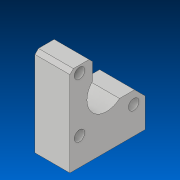
# Autodesk Inventor part: y-stepper-mount
Saved by Autodesk Inventor 2021 (Build 250183000, 183)
## iProperties
RuleStatus: InUse
Created: 2019-07-31
Part Number: y-stepper-mount
Material: Všeobecné
Document SubType Name: Modeling
Designer: Robert Turinský
Density: 1 g/cm^3
Appearance: Výchozí
Author: Robert Turinský
Autodesk Inventor part; units mm, degrees
ref_plane "XY Plane" through (0, 0, 0) normal (0, 0, 1) x (1, 0, 0)
sketch "Náčrt1" plane through (0, 0, 0) normal (0, 0, 1) x (1, 0, 0)
  line L0 (0, -49.6) -> (0, 14.1) projected
  line L1 (-71.6, 0) -> (163.6, 0) projected
  arc A0 (0.375, -4.0577) -> (-0.375, -4.0577) centre (0, 0) ccw
  arc A1 (120.375, -4.0577) -> (119.625, -4.0577) centre (120, 0) ccw
  line L2 (5, 5) -> (-5, 5)
  line L3 (-5, 5) -> (-8.1754, -0.5)
  line L4 (-8.1754, -0.5) -> (-35.5, -0.5)
  line L5 (-35.5, -0.5) -> (-38, -3)
  line L6 (-38, -3) -> (-38, -38)
  line L7 (-38, -38) -> (-35.5, -40.5)
  line L8 (-35.5, -40.5) -> (114, -40.5)
  line L9 (114, -40.5) -> (130, -24.5)
  line L10 (130, -24.5) -> (130, -3.6603)
  line L11 (130, -3.6603) -> (125, 5)
  line L12 (125, 5) -> (115, 5)
  line L13 (115, 5) -> (111.8246, -0.5)
  line L14 (111.8246, -0.5) -> (8.1754, -0.5)
  line L15 (8.1754, -0.5) -> (5, 5)
  circle A2 centre (87.45, -12.35) radius 2.65
  circle A3 centre (110.7, -35.6) radius 2.65
  circle A4 centre (-32.55, -12.35) radius 2.65
  circle A5 centre (-9.3, -35.6) radius 2.65
  line L16 (119.625, -4.0577) -> (119.625, -12)
  line L17 (119.625, -12) -> (120.375, -12)
  line L18 (120.375, -12) -> (120.375, -4.0577)
  line L19 (-0.375, -4.0577) -> (-0.375, -12)
  line L20 (-0.375, -12) -> (0.375, -12)
  line L21 (0.375, -12) -> (0.375, -4.0577)
  point P0 (120, 5)
  point P1 (0, 5)
  dimension "d0" = 8.15
  dimension "d1" = 120
  dimension "d2" = 0.5
  dimension "d3" = 5.5
  dimension "d4" = 10
  dimension "d5" = 60
  dimension "d6" = 2.5
  dimension "d7" = 2.5
  dimension "d8" = 38
  dimension "d9" = 40.5
  dimension "d10" = 168
  dimension "d11" = 16
  dimension "d12" = 5.3
  dimension "d13" = 5.45
  dimension "d14" = 28.15
  dimension "d15" = 23.25
  dimension "d16" = 23.25
  dimension "d17" = 23.25
  dimension "d18" = 120
  dimension "d25" = 0.75
  dimension "d26" = 12
  constraints: 40 end point, 7 equal length, 6 centre point, 6 parallel, 5 point on line, 4 equal radius, 4 point on circle, 3 perpendicular, 2 horizontal alignment, 2 midpoint, 2 vertical, 2 vertical alignment, 1 coincident, 1 collinear, 1 horizontal
  measures "d0" diameter of A0
  measures "d1" distance of A0.centre A1.centre
  measures "d2" distance between parallel lines of L1 L4
  measures "d3" distance between parallel lines of L4 L2
  measures "d4" distance of L2.start L2.end
  measures "d5" angle of L2 L3
  measures "d6" horizontal distance of L4.end L5.end
  measures "d7" horizontal distance of L4.end L5.end
  measures "d8" distance between parallel lines of L6 L0
  measures "d9" distance between parallel lines of L8 L1
  measures "d10" distance between parallel lines of L6 L10
  measures "d11" horizontal distance of L8.end L9.end
  measures "d12" diameter of A2
  measures "d13" distance from line of L6 A4.centre
  measures "d14" distance from line of L8 A4.centre
  measures "d15" horizontal distance of A5.centre A4.centre
  measures "d16" horizontal distance of A4.centre A5.centre
  measures "d17" horizontal distance of A2.centre A3.centre
  measures "d18" distance of A4.centre A2.centre
  measures "d25" distance between parallel lines of L16 L18
  measures "d26" distance between parallel lines of L17 L1
extrude "Vysunutí1" add sketch "Náčrt1" along normal blind 11.95 contours L8 L7 L6 L5 L4 L3 L1 A0 L19 L20 L0 | L0 L20 L21 A0 L1 L15 L14 L13 A1 L16 L17 L18 L11 L10 L9 L8 | A0 L1 L3 L2 L0 | L0 L2 L15 L1 A0 | L1 A1 L13 L12 L11
extrude "Vysunutí2" [suppressed]
ref_plane "Pracovní rovina1" through (50, 0, 0) normal (1, 0, 0) x (0, 1, 0)
sketch "Náčrt3" plane through (50, 0, 0) normal (1, 0, 0) x (0, 1, 0)
  line L0 (-0.5, 0) -> (-0.5, 11.95) projected
  line L1 (-48.9, 0) -> (9.9, 0) projected
  line L2 (0, -53.99) -> (0, 22.94) projected
  circle A0 centre (-18, -21) radius 11.25
  line L3 (-0.5, 0) -> (1.5, -2)
  line L4 (1.5, -2) -> (1.5, -11)
  line L5 (1.5, -11) -> (-0.5, -13)
  line L6 (-0.5, -13) -> (-10.0904, -13)
  line L7 (-26.5, -28.3697) -> (-26.5, -37)
  line L8 (-26.5, -37) -> (-32.5, -43)
  line L9 (-32.5, -43) -> (-36, -43)
  line L10 (-36, -43) -> (-39, -40)
  line L11 (-39, -40) -> (-40.5, -27)
  line L12 (-40.5, -27) -> (-40.5, 0)
  line L13 (-0.5, 0) -> (-0.5, 11.95) projected
  line L14 (-40.5, 0) -> (-0.5, 0)
  line L15 (-40.5, 0) -> (-40.5, 11.95) projected
  circle A1 centre (-2.5, -5.5) radius 1.7
  circle A2 centre (-33.5, -5.5) radius 1.7
  circle A3 centre (-33.5, -36.5) radius 1.7
  point P0 (0, 0)
  dimension "d28" = 22.5
  dimension "d29" = 21
  dimension "d30" = 18
  dimension "d31" = 8
  dimension "d32" = 19.5
  dimension "d33" = 45
  dimension "d34" = 8.5
  dimension "d35" = 6
  dimension "d36" = 22
  dimension "d37" = 3
  dimension "d38" = 13
  dimension "d39" = 1.5
  dimension "d40" = 3.4
  dimension "d41" = 31
  dimension "d42" = 31
  dimension "d43" = 15.5
  dimension "d44" = 15.5
  constraints: 22 end point, 5 perpendicular, 4 centre point, 3 vertical, 2 equal radius, 2 horizontal, 2 point on circle, 2 point on line, 1 horizontal alignment, 1 vertical alignment
  measures "d28" diameter of A0
  measures "d29" distance from line of L1 A0.centre
  measures "d30" distance from line of L2 A0.centre
  measures "d31" distance from line of A0.centre L6
  measures "d32" distance from line of A0.centre L4
  measures "d33" angle of L1 L3
  measures "d34" distance from line of L7 A0.centre
  measures "d35" horizontal distance of L7.end L8.end
  measures "d36" distance from line of A0.centre L9
  measures "d37" horizontal distance of L9.end L10.end
  measures "d38" vertical distance of L10.end L11.end
  measures "d39" horizontal distance of L10.end L11.end
  measures "d40" diameter of A1
  measures "d41" distance of A2.centre A1.centre
  measures "d42" distance of A3.centre A2.centre
  measures "d43" horizontal distance of A0.centre A2.centre
  measures "d44" horizontal distance of A0.centre A2.centre
extrude "Vysunutí4" add sketch "Náčrt3" along normal blind 20 contours L1 L3 L2 L5 L6 A0 L7 L8 L9 L10 L11 L12 | L3 L4 L5 L2
sketch "Náčrt5" plane through (70, 0, 0) normal (1, 0, 0) x (0, 0, -1)
  point P0 (0, 0)
  point P1 (5.5, -2.5)
  point P2 (5.5, -33.5)
  point P3 (36.5, -33.5)
hole "Díra1" at (70, -2.5, -5.5) at (70, -33.5, -5.5) at (70, -33.5, -36.5) direction (-1, 0, 0) diameter 3.4 end through all counterbore diameter 6 counterbore depth 11
ref_plane "Pracovní rovina2" through (0, -23.975, 0) normal (0, 1, 0) x (-1, 0, 0)
ref_plane "Pracovní rovina4" through (57.65, -2.5, -5.5) normal (1, 0, 0) x (0, 0, -1)
ref_plane "Pracovní rovina5" through (0, 0, 5.975) normal (0, 0, 1) x (1, 0, 0)
ref_plane "Pracovní rovina7" through (0, -33.975, 0) normal (0, 1, 0) x (-1, 0, 0)
sketch "Sketch19" plane through (130, -24.5, 0) normal (1, 0, 0) x (0, 0, -1)
  line L0 (0, -16) -> (-11.95, -16) projected
  line L1 (0, 29.5) -> (-11.95, 29.5) projected
  line L2 (-11.95, 20.7058) -> (-11.95, 0.2071) projected
  line L3 (0, 0) -> (0, 20.8397) projected
  line L4 (0, 29.5) -> (0, 24) projected
  line L5 (0, 29.5) -> (-11.95, 29.5)
  line L6 (-11.95, 29.5) -> (-11.95, -16)
  line L7 (0, -16) -> (-11.95, -16) projected
  line L8 (-11.95, -16) -> (0, -16)
  line L9 (0, -16) -> (0, 29.5)
  point P0 (0, 24.5)
  point P1 (-10.5763, -16)
  point P2 (-10.5763, 29.5)
  point P3 (-10.5763, 29.5)
  point P4 (-10.5763, -16)
  constraints: 9 end point, 2 perpendicular, 1 collinear
extrude "Extrusion20" cut sketch "Sketch19" against normal through all
sketch "Sketch20" plane through (50, 0, 0) normal (-1, 0, 0) x (0, 0, 1)
  line L0 (-40, -39) -> (-43, -36) projected
  line L1 (-43, -36) -> (-43, -49.2119)
  line L2 (-43, -49.2119) -> (0, -49.2119)
  line L3 (0, -40.5) -> (-27, -40.5) projected
  line L4 (0, -49.2119) -> (0, -40.5)
  line L5 (-27, -40.5) -> (-40, -39) projected
  point P0 (0, 0)
  constraints: 6 end point, 2 perpendicular, 1 vertical
extrude "Extrusion21" add sketch "Sketch20" against normal up to surface (20 mm away)
equation "\"d7\" = d6"
equation "\"d16\" = d15"
equation "\"d17\" = d15"
equation "\"d42\" = d41"
equation "\"d43\" = 0.5 * d41"
equation "\"d44\" = 0.5 * d41"
